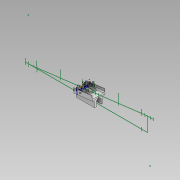
# Autodesk Inventor part: Slope_Middle
Saved by Autodesk Inventor 2021 (Build 250183000, 183)
## iProperties
Created: 2021-03-11
Part Number: Slope_Middle
Material: 一般
Document SubType Name: Modeling
Designer: kumagai
Density: 1 g/cm^3
Appearance: 既定
Author: kumagai
Autodesk Inventor part; units mm, degrees
ref_plane "YZ Plane" through (0, 0, 0) normal (1, 0, 0) x (0, 1, 0)
ref_plane "XZ Plane" through (0, 0, 0) normal (0, 1, 0) x (-1, 0, 0)
ref_plane "XY Plane" through (0, 0, 0) normal (0, 0, 1) x (1, 0, 0)
derived "SlopeProfile.ipt"
sketch "スケッチ1" plane through (0, 0, 0) normal (0, 0, 1) x (1, 0, 0)
  line L0 (0, 14) -> (0, -14)
  line L1 (-14, 0) -> (14, 0)
  line L2 (-268.75, 0) -> (268.75, 0)
  line L3 (-268.75, 0) -> (268.75, 66)
  line L4 (268.75, 66) -> (268.75, 0)
  line L5 (-31.5879, 61.457) -> (-25.6465, 13.0705)
  line L6 (-134.375, 50.6657) -> (-134.375, 8.5939)
  line L7 (23.2129, 72.7486) -> (28.7067, 28.0077)
  line L8 (-244.2356, 29.1492) -> (-240.1953, -3.7549)
  line L9 (134.375, 89.7324) -> (134.375, 45.3233)
  line L10 (239.1121, 78.5758) -> (241.9591, 55.3901)
  line L11 (-27.6764, 5.7379) -> (-27.6764, -11.9933)
  line L12 (27.6764, 6.5088) -> (27.6764, -13.0212)
  line L13 (-268.75, 0) -> (-295.625, 0)
  line L14 (268.75, 66) -> (295.625, 66)
  line L15 (241.0736, 6.6999) -> (241.0736, -9.2827)
  line L16 (-241.0736, -7.7427) -> (-241.0736, -14.414)
  arc A0 (-280.625, 0) -> (-256.9635, 1.4473) centre (-280.625, 194.1449) ccw
  line L17 (-256.3082, 4.3915) -> (-255.7778, 0.0713)
  line L18 (-280.625, 8.6126) -> (-280.625, -11.6883)
  line L19 (-295.625, 14.7784) -> (-295.625, -11.568)
  line L20 (255.3892, 69.0933) -> (256.9398, 56.465)
  line L21 (280.625, 71.1514) -> (280.625, 58.4982)
  line L22 (295.625, 71.9522) -> (295.625, 60.0478)
  arc A1 (280.625, 66) -> (256.9635, 64.5527) centre (280.625, -128.1449) ccw
  line L23 (-13.2739, 35.3851) -> (-12.039, 25.3288)
  line L24 (-43.1495, 32.5373) -> (-41.4451, 18.6566)
  line L25 (12.2235, 39.1691) -> (13.7539, 26.7059)
  line L26 (41.8424, 44.108) -> (43.6336, 29.5201)
  point P0 (0, 0)
  point P1 (-241.0736, 3.3984)
  point P2 (-27.6764, 29.6016)
  point P3 (27.6764, 36.3984)
  point P4 (241.0736, 62.6016)
  point P5 (134.375, 49.5)
  point P6 (-134.375, 16.5)
ref_plane "作業平面1" through (-27.6764, 29.6016, 0) normal (0.9925454, 0.1218753, 0) x (-0.1218753, 0.9925454, 0)
sketch "スケッチ2" plane through (-27.6764, 29.6016, 0) normal (0.9925454, 0.1218753, 0) x (-0.1218753, 0.9925454, 0)
  line L0 (-5.2, 19) -> (-5.2, -19)
  line L1 (-5.2, -19) -> (3.2, -19)
  line L2 (3.2, -19) -> (3.2, -17)
  line L3 (3.2, -17) -> (0, -17)
  line L4 (0, -17) -> (0, -9.3)
  line L5 (0, -9.3) -> (3.2, -9.3)
  line L6 (3.2, -9.3) -> (3.2, -6.9)
  line L7 (3.2, -6.9) -> (0, -6.9)
  line L8 (0, -6.9) -> (0, 6.9)
  line L9 (0, 6.9) -> (3.2, 6.9)
  line L10 (3.2, 6.9) -> (3.2, 9.3)
  line L11 (3.2, 9.3) -> (0, 9.3)
  line L12 (0, 9.3) -> (0, 17)
  line L13 (0, 17) -> (3.2, 17)
  line L14 (3.2, 17) -> (3.2, 19)
  line L15 (3.2, 19) -> (-5.2, 19)
  line L16 (32.0946, 0) -> (-16.6552, 0) projected
  line L17 (-5.2, 27.5) -> (-5.2, -27.5)
  line L18 (-5.2, -27.5) -> (9, -27.5)
  line L19 (9, -27.5) -> (9, -29.5)
  line L20 (9, -29.5) -> (-11, -29.5)
  line L21 (-11, -29.5) -> (-11, 29.5)
  line L22 (-11, 29.5) -> (9, 29.5)
  line L23 (9, 29.5) -> (9, 27.5)
  line L24 (9, 27.5) -> (-5.2, 27.5)
  point P0 (-32.754, 0)
  point P1 (0, 0)
  point P2 (0, 0)
  point P3 (0, 0)
  dimension "d25" = 8.4
  dimension "d26" = 3.2
  dimension "d27" = 38
  dimension "d28" = 2
  dimension "d29" = 2.4
  dimension "d30" = 18.6
  dimension "d31" = 20
  dimension "d32" = 5.8
  dimension "d33" = 5.8
  dimension "d34" = 59
  dimension "d35" = 2
  constraints: 49 end point, 17 perpendicular, 10 point on line, 2 collinear, 2 vertical, 1 midpoint, 6 other
  measures "d25" distance between parallel lines of L0 L2
  measures "d26" distance between parallel lines of L4 L2
  measures "d27" distance between parallel lines of L1 L15
  measures "d28" distance between parallel lines of L15 L13
  measures "d29" distance between parallel lines of L9 L11
  measures "d30" distance between parallel lines of L5 L11
  measures "d31" distance between parallel lines of L21 L19
  measures "d32" distance between parallel lines of L19 L2
  measures "d33" distance between parallel lines of L21 L17
  measures "d34" distance between parallel lines of L20 L22
  measures "d35" distance between parallel lines of L22 L24
extrude "押し出し1" add sketch "スケッチ2" along normal blind 60 contours L15 L14 L13 L12 L11 L10 L9 L8 L16 L0 | L16 L8 L7 L6 L5 L4 L3 L2 L1 L0
sketch "スケッチ3" plane through (0, 0, 0) normal (0, 0, 1) x (1, 0, 0)
  line L0 (-268.75, 0) -> (268.75, 66) projected
  line L1 (12.2235, 39.1691) -> (13.7539, 26.7059) projected
  line L2 (-13.2739, 35.3851) -> (-12.039, 25.3288) projected
  line L3 (-14.0069, 41.3552) -> (-11.5694, 21.5043)
  line L4 (-11.5694, 21.5043) -> (14.0069, 24.6448)
  line L5 (14.0069, 24.6448) -> (11.5694, 44.4957)
  line L6 (11.5694, 44.4957) -> (-14.0069, 41.3552)
  line L7 (-45.0021, 47.6244) -> (-40.127, 7.9226)
  line L8 (-40.127, 7.9226) -> (45.0021, 18.3756)
  line L9 (45.0021, 18.3756) -> (40.127, 58.0774)
  line L10 (40.127, 58.0774) -> (-45.0021, 47.6244)
  line L11 (-31.5879, 61.457) -> (-25.6465, 13.0705) projected
  line L12 (23.2129, 72.7486) -> (28.7067, 28.0077) projected
  line L13 (-67.2905, 65.0378) -> (-57.5404, -14.3659)
  line L14 (-57.5404, -14.3659) -> (67.2905, 0.9622)
  line L15 (67.2905, 0.9622) -> (57.5404, 80.3659)
  line L16 (57.5404, 80.3659) -> (-67.2905, 65.0378)
  point P0 (0, 0)
  dimension "d38" = 20
  dimension "d39" = 10
  dimension "d40" = 10
  dimension "d49" = 15
  dimension "d50" = 15
  dimension "d51" = 20
  constraints: 24 end point, 5 perpendicular, 3 parallel, 2 collinear, 4 other
  measures "d38" distance between parallel lines of L4 L6
  measures "d39" distance between parallel lines of L6 L10
  measures "d40" distance between parallel lines of L8 L4
  measures "d49" distance between parallel lines of L11 L7
  measures "d50" distance between parallel lines of L9 L12
  measures "d51" distance between parallel lines of L16 L10
extrude "押し出し2" cut sketch "スケッチ3" along normal through all both and the other way through all contours L7 L10 L11 L0 | L0 L2 L3 L4 L5 L1 L9 L8 L7 | L11 L10 L12 L0 L1 L5 L6 L3 L2 | L10 L9 L0 L12
extrude "押し出し3" add sketch "スケッチ2" along normal blind 90 and the other way blind 30 contours L0 L16 L21 L22 L23 L24 L17 | L0 L17 L18 L19 L20 L21 L16
extrude "押し出し4" cut sketch "スケッチ3" against normal through all both and the other way through all contours L13 L16 L15 L0 L9 L10 L7 | L0 L7 L8 L9 L15 L14 L13
sketch "スケッチ4" plane through (-27.6764, 29.6016, 0) normal (0.9925454, 0.1218753, 0) x (-0.1218753, 0.9925454, 0)
  line L0 (-11, -29.5) -> (-11, 29.5) projected
  line L1 (9, 29.5) -> (-11, 29.5) projected
  line L2 (-11, 29.5) -> (-20.0203, 18.75)
  line L3 (-20.0203, 18.75) -> (-51, 18.75)
  line L4 (-51, 18.75) -> (-51, 10.75)
  line L5 (-51, 10.75) -> (-20.0203, 10.75)
  line L6 (-20.0203, 10.75) -> (-11, 0)
  line L7 (-20.0203, -10.75) -> (-51, -10.75)
  line L8 (-51, -10.75) -> (-51, -18.75)
  line L9 (-51, -18.75) -> (-20.0203, -18.75)
  line L10 (-11, 29.5) -> (-11, -29.5) projected
  line L11 (-20.0203, -18.75) -> (-11, -29.5)
  line L12 (-11, -29.5) -> (-11, 0)
  line L13 (-20.0203, -10.75) -> (-11, 0)
  line L14 (-11, 0) -> (-11, 29.5)
  line L15 (32.0946, 0) -> (-16.6552, 0) projected
  point P0 (-32.754, 0)
  dimension "d54" = 40
  dimension "d55" = 40
  dimension "d56" = 8
  dimension "d57" = 40
  constraints: 24 end point, 3 parallel, 3 perpendicular, 2 point on line, 1 collinear, 1 midpoint, 1 vertical alignment, 4 other
  measures "d54" angle of L0 L2
  measures "d55" angle of L0 L6
  measures "d56" distance between parallel lines of L5 L3
  measures "d57" distance between parallel lines of L0 L4
extrude "押し出し5" add sketch "スケッチ4" along normal blind 90 and the other way blind 30
sketch "スケッチ5" plane through (0, 0, 0) normal (0, 0, 1) x (1, 0, 0)
  line L0 (-268.75, 0) -> (268.75, 0) projected
  line L1 (-41.2239, 16.8555) -> (43.9052, 27.3085)
  line L2 (43.9052, 27.3085) -> (43.9052, -5.2)
  line L3 (43.9052, -5.2) -> (-41.2239, -5.2)
  line L4 (-41.2239, -5.2) -> (-41.2239, 16.8555)
  line L5 (-268.75, 0) -> (268.75, 66) projected
  line L6 (-56.1121, 15.0273) -> (-41.2239, 16.8555) projected
  line L7 (-41.2239, 16.8555) -> (-71.0003, 13.1992)
  line L8 (-71.0003, 13.1992) -> (-64.9065, -36.4281)
  line L9 (-64.9065, -36.4281) -> (79.7753, -18.6625)
  line L10 (79.7753, -18.6625) -> (73.6815, 30.9648)
  line L11 (-41.2239, 16.8555) -> (43.9052, 27.3085) projected
  line L12 (73.6815, 30.9648) -> (43.9052, 27.3085)
  point P0 (0, 0)
  point P1 (43.9052, 0)
  point P2 (-41.2239, 0)
  point P3 (-69.3795, 0)
  point P4 (77.4837, 0)
  dimension "d62" = 50
  dimension "d63" = 30
  dimension "d64" = 30
  dimension "d67" = 5.2
  constraints: 18 end point, 3 parallel, 3 perpendicular, 2 collinear
  measures "d62" distance between parallel lines of L9 L7
  measures "d63" distance from line of L1.start L8
  measures "d64" distance from line of L10 L1.end
  measures "d67" distance between parallel lines of L3 L0
extrude "押し出し6" cut sketch "スケッチ5" against normal through all both and the other way through all contours L8 L7 L6 L4 L0 | L0 L4 L3 L2 L10 L9 L8 | L2 L12 L10 L0
chamfer "面取り1" distance 5 angle 45 2 edges at (0.6338, 27.8388, -27.5) (0.6338, 27.8388, 27.5)
equation "\"d25\" = RailHeight"
equation "\"d26\" = RailDepth"
equation "\"d27\" = RailWidth"
equation "\"d28\" = OuterWall"
equation "\"d29\" = InnerWall"
equation "\"d30\" = InsideWidth"
equation "\"d32\" = d33"
equation "\"d67\" = RailHeight - RailDepth"
equation "\"RailHeight\" = 8.4"
equation "\"RailDepth\" = 3.2"
equation "\"RailWidth\" = 38"
equation "\"OuterWall\" = 2"
equation "\"InnerWall\" = 2.4"
equation "\"InsideWidth\" = 18.6"
